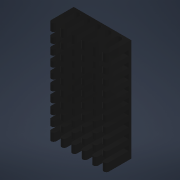
# Autodesk Inventor part: heatsink
Saved by Autodesk Inventor 2021 (Build 250183000, 183)
## iProperties
Created: 2021-01-23
Part Number: heatsink
Material: Generic
Document SubType Name: Modeling
Designer: User
Density: 1 g/cm^3
Appearance: Iron Black
Author: User
Autodesk Inventor part; units mm, degrees
ref_plane "YZ Plane" through (0, 0, 0) normal (1, 0, 0) x (0, 1, 0)
ref_plane "XZ Plane" through (0, 0, 0) normal (0, 1, 0) x (-1, 0, 0)
ref_plane "XY Plane" through (0, 0, 0) normal (0, 0, 1) x (1, 0, 0)
sketch "Sketch1" plane through (0, 0, 0) normal (0, 0, 1) x (1, 0, 0)
  line L0 (12.5, 21) -> (12.5, -21) projected
  line L1 (-12.5, 21) -> (12.5, 21) projected
  line L2 (-12.5, -21) -> (-12.5, 21) projected
  line L3 (12.5, -21) -> (-12.5, -21) projected
  line L4 (-11.5, 20.5) -> (11.5, 20.5)
  line L5 (11.5, 20.5) -> (11.5, -20.5)
  line L6 (11.5, -20.5) -> (-11.5, -20.5)
  line L7 (-11.5, -20.5) -> (-11.5, 20.5)
  line L8 (-11.5, 20.5) -> (11.5, -20.5) construction
  line L9 (11.5, 20.5) -> (-11.5, -20.5) construction
  point P0 (0, 0)
  dimension "d0" = 23
  dimension "d1" = 41
  constraints: 12 end point, 2 midpoint, 2 parallel, 1 horizontal, 1 perpendicular
  measures "d0" distance of L5.end L6.end
  measures "d1" distance of L4.end L5.end
extrude "Extrusion1" add sketch "Sketch1" along normal blind 10 contours L4 L5 L6 L7
sketch "Sketch3" plane through (-11.5, 20.5, 0) normal (0, 1, 0) x (1, 0, 0)
  line L0 (0, -10) -> (23, -10) projected
  line L1 (23, -10) -> (21, -10)
  line L2 (21, -10) -> (21, -1)
  line L3 (21, -1) -> (23, -1)
  line L4 (23, -1) -> (23, -10)
  line L5 (16.8, -10) -> (16.8, -1)
  line L6 (18.8, -10) -> (16.8, -10)
  line L7 (18.8, -1) -> (18.8, -10)
  line L8 (16.8, -1) -> (18.8, -1)
  line L9 (12.6, -10) -> (12.6, -1)
  line L10 (14.6, -10) -> (12.6, -10)
  line L11 (14.6, -1) -> (14.6, -10)
  line L12 (12.6, -1) -> (14.6, -1)
  line L13 (8.4, -10) -> (8.4, -1)
  line L14 (10.4, -10) -> (8.4, -10)
  line L15 (10.4, -1) -> (10.4, -10)
  line L16 (8.4, -1) -> (10.4, -1)
  line L17 (4.2, -10) -> (4.2, -1)
  line L18 (6.2, -10) -> (4.2, -10)
  line L19 (6.2, -1) -> (6.2, -10)
  line L20 (4.2, -1) -> (6.2, -1)
  line L21 (0, -10) -> (0, -1)
  line L22 (2, -10) -> (0, -10)
  line L23 (2, -1) -> (2, -10)
  line L24 (0, -1) -> (2, -1)
  line L25 (23, 0) -> (0, 0) projected
  line L26 (23, -1) -> (0, -1)
  line L27 (0, 0) -> (23, 0) projected
  point P0 (11.5, 0)
  point P1 (4.2, -1)
  point P2 (8.4, -1)
  point P3 (12.6, -1)
  point P4 (16.8, -1)
  point P5 (21, -1)
  dimension "d17" = 4.2
  dimension "d22" = 2
  dimension "d23" = 23
  dimension "d26" = 1
  constraints: 50 end point, 3 parallel, 2 horizontal, 1 perpendicular, 40 other
  measures "d17" distance of L1.end L5.start
  measures "d22" distance between parallel lines of L4 L2
  measures "d23" distance of L0.start L0.end
  measures "d26" distance between parallel lines of L25 L3
extrude "Extrusion2" cut sketch "Sketch3" against normal up to surface (41 mm away) contours L23 L26 L17 L0 | L19 L26 L13 L0 | L15 L26 L9 L0 | L11 L26 L5 L0 | L7 L26 L2 L0
sketch "Sketch2" plane through (-11.5, -20.5, 0) normal (-1, 0, 0) x (0, 0, 1)
  line L0 (10, 0) -> (10, 41) projected
  line L1 (10, 38) -> (1, 38)
  line L2 (1, 38) -> (1, 36)
  line L3 (1, 36) -> (10, 36)
  line L4 (10, 36) -> (10, 38)
  line L5 (10, 33.8889) -> (1, 33.8889)
  line L6 (1, 31.8889) -> (10, 31.8889)
  line L7 (10, 31.8889) -> (10, 33.8889)
  line L8 (1, 33.8889) -> (1, 31.8889)
  line L9 (10, 29.7778) -> (1, 29.7778)
  line L10 (1, 27.7778) -> (10, 27.7778)
  line L11 (10, 27.7778) -> (10, 29.7778)
  line L12 (1, 29.7778) -> (1, 27.7778)
  line L13 (10, 25.6667) -> (1, 25.6667)
  line L14 (1, 23.6667) -> (10, 23.6667)
  line L15 (10, 23.6667) -> (10, 25.6667)
  line L16 (1, 25.6667) -> (1, 23.6667)
  line L17 (10, 21.5556) -> (1, 21.5556)
  line L18 (1, 19.5556) -> (10, 19.5556)
  line L19 (10, 19.5556) -> (10, 21.5556)
  line L20 (1, 21.5556) -> (1, 19.5556)
  line L21 (10, 17.4444) -> (1, 17.4444)
  line L22 (1, 15.4444) -> (10, 15.4444)
  line L23 (10, 15.4444) -> (10, 17.4444)
  line L24 (1, 17.4444) -> (1, 15.4444)
  line L25 (10, 13.3333) -> (1, 13.3333)
  line L26 (1, 11.3333) -> (10, 11.3333)
  line L27 (10, 11.3333) -> (10, 13.3333)
  line L28 (1, 13.3333) -> (1, 11.3333)
  line L29 (10, 9.2222) -> (1, 9.2222)
  line L30 (1, 7.2222) -> (10, 7.2222)
  line L31 (10, 7.2222) -> (10, 9.2222)
  line L32 (1, 9.2222) -> (1, 7.2222)
  line L33 (10, 5.1111) -> (1, 5.1111)
  line L34 (1, 3.1111) -> (10, 3.1111)
  line L35 (10, 3.1111) -> (10, 5.1111)
  line L36 (1, 5.1111) -> (1, 3.1111)
  line L37 (0, 0) -> (10, 0) projected
  line L38 (0, 41) -> (10, 41) projected
  line L39 (0, 41) -> (0, 0) projected
  point P0 (0, 20.5)
  point P1 (10, 3.1111)
  point P2 (10, 5.1111)
  point P3 (10, 7.2222)
  point P4 (10, 9.2222)
  point P5 (10, 11.3333)
  point P6 (10, 13.3333)
  point P7 (10, 15.4444)
  point P8 (10, 17.4444)
  point P9 (10, 19.5556)
  point P10 (10, 23.6667)
  point P11 (10, 27.7778)
  point P12 (10, 31.8889)
  point P13 (10, 36)
  dimension "d4" = 2
  dimension "d7" = 4.1111
  dimension "d13" = 3.1111
  dimension "d14" = 41
  dimension "d30" = 3
  dimension "d31" = 1
  constraints: 72 end point, 32 vertical alignment, 17 parallel, 16 collinear, 1 horizontal, 1 perpendicular, 3 other
  measures "d4" distance of L2.end L1.end
  measures "d7" distance of L1.start L5.start
  measures "d13" distance between parallel lines of L37 L34
  measures "d14" distance of L37.end L38.end
  measures "d30" distance between parallel lines of L38 L1
  measures "d31" distance between parallel lines of L39 L2
fillet "Fillet1" radius 1 22 edges at (9.5, 0, 1) (7.3, 0, 1) (5.3, 0, 1) (3.1, 0, 1) (1.1, 0, 1) (-1.1, 0, 1) (-3.1, 0, 1) (-5.3, 0, 1) (-7.3, 0, 1) (-9.5, 0, 1) (11.5, 0, 10) (9.5, 0, 10) (7.3, 0, 10) (5.3, 0, 10) (3.1, 0, 10) (1.1, 0, 10) (-1.1, 0, 10) (-3.1, 0, 10) (-5.3, 0, 10) (-7.3, 0, 10) (-9.5, 0, 10) (-11.5, 0, 10)
extrude "Extrusion3" cut sketch "Sketch2" against normal up to surface (23 mm away) contours L34 L36 L33 L0 | L30 L32 L29 L0 | L0 L3 L2 L1 | L26 L28 L25 L0 | L0 L6 L8 L5 | L22 L24 L21 L0 | L0 L10 L12 L9 | L18 L20 L17 L0 | L0 L14 L16 L13
equation "\"d17\" = -0.2 * d22 + 0.2 * d23"
equation "\"d7\" = 0.111111 * d4 + 0.111111 * d14 - 0.222222 * d12"
equation "\"d12\" = 3"
body "Solid1"
